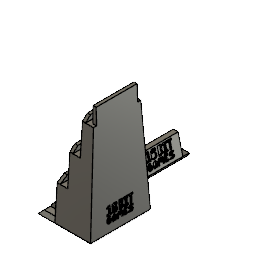
Nintendo DS Stand v8 (Autodesk Fusion 360 design; units mm, degrees)
Autodesk Fusion 360 part; units mm, degrees
(part 1 of 2)
sketch "Sketch1" plane through (0, 0, 0) normal (1, 0, 0) x (0, 0, -1)
  circle A0 centre (0, 0) radius 60
  line L0 (0.167, -59.9998) -> (20.167, -59.9998)
  line L1 (20.167, -59.9998) -> (20.167, -55)
  line L2 (20.167, -55) -> (-19.833, -55)
  line L3 (-19.833, -55) -> (-19.833, -59.9998)
  line L4 (-19.833, -59.9998) -> (20.167, -59.9998)
  line L5 (20.167, -59.9998) -> (20.167, -55)
  line L6 (20.167, -59.9998) -> (-19.833, -59.9998)
  line L7 (-19.833, -59.9998) -> (-19.833, -61.9998)
  line L8 (-19.833, -61.9998) -> (20.167, -61.9998)
  line L9 (20.167, -61.9998) -> (20.167, -59.9998)
  dimension "d1" = 120
  dimension "d2" = 20
  dimension "d3" = 40
  dimension "d4" = 2
  constraint coincident A0.centre origin
  constraint coincident A0 L0.start
  constraint horizontal L0
  constraint perpendicular L0 L1
  constraint horizontal L2
  constraint vertical L3
  constraint horizontal L4
  constraint vertical L5
  constraint horizontal L6
  constraint vertical L7
  constraint horizontal L8
  constraint vertical L9
  measures "d1" diameter of A0
  measures "d2" distance of L0.start L0.end
  measures "d3" distance of L1.end L2.end
  measures "d4" distance of L0.end L8.end
sketch "Sketch4" plane through (0, 0, 0) normal (1, 0, 0) x (0, 0, -1)
  line L0 (0, 0) -> (13, 0)
  line L1 (13, 0) -> (13, 10)
  line L2 (13, 10) -> (-13, 10)
  line L3 (-13, 10) -> (-13, 0)
  line L4 (-13, 0) -> (13, 0)
  line L5 (13, 0) -> (13, 10)
  dimension "d21" = 13
  dimension "d22" = 10
  dimension "d23" = 26
  dimension "d24" = 10
  constraint coincident L0.start origin
  constraint horizontal L0
  constraint perpendicular L0 L1
  constraint horizontal L2
  constraint vertical L3
  constraint horizontal L4
  constraint vertical L5
  measures "d21" distance of L0.start L0.end
  measures "d22" distance of L0.end L1.end
  measures "d23" distance of L1.end L2.end
  measures "d24" distance of L1.end L0.end
extrude "Extrude4" add sketch "Sketch4" along normal blind 2 makes body 1
sketch "Sketch5" plane through (2, 0, 0) normal (1, 0, 0) x (0, 0, -1)
  line L0 (13, 0) -> (13, 10)
  line L1 (13, 10) -> (-13, 10)
  line L2 (-13, 10) -> (-13, 0)
  line L3 (-13, 0) -> (13, 0)
  line L4 (-13, 0) -> (13, 0)
  line L5 (13, 0) -> (13, -2)
  line L6 (13, -2) -> (-13, -2)
  line L7 (-13, -2) -> (-13, 0)
  dimension "d27" = 2
  constraint horizontal L4
  constraint vertical L5
  constraint horizontal L6
  constraint vertical L7
  constraint coincident L2.end L3.start
  measures "d27" distance of L2.end L6.end
extrude "Extrude5" add sketch "Sketch5" along normal blind 2 separate body contours L3 L4 L5 L6 L7 makes body 2
extrude "Extrude6" add 1 faces at (2, -1.3333, -4.3333) along direction (-1, 0, 0) blind 3 on bodies 2 bodies 2 1
sketch "Sketch6" plane through (0, 0, 0) normal (0, 1, 0) x (-1, 0, 0)
  line L0 (0, 13) -> (0, -13)
  line L1 (0, -13) -> (1, -13)
  line L2 (1, -13) -> (1, 13)
  line L3 (1, 13) -> (0, 13)
  line L4 (1, 13) -> (3, 13)
  line L5 (3, 13) -> (3, -13)
  line L6 (3, -13) -> (1, -13)
  line L7 (1, -13) -> (1, 13)
  dimension "d32" = 2
  constraint horizontal L4
  constraint vertical L5
  constraint horizontal L6
  constraint vertical L7
  constraint coincident L2.end L3.start
  measures "d32" distance of L2.end L4.end
extrude "Extrude7" add sketch "Sketch6" along normal blind 3 separate body contours L2 L4 L5 L6 L7 makes body 3
extrude "Extrude8" add 1 faces at (-1, -1.3333, -4.3333) along direction (-1, 0, 0) blind 4 on bodies 2 bodies 2 3
sketch "Sketch7" plane through (0, 0, 13) normal (0, 0, 1) x (1, 0, 0)
  line L0 (-5, -2) -> (4, -2)
  line L1 (4, -2) -> (4, 0)
  line L2 (4, 0) -> (2, 0)
  line L3 (2, 0) -> (2, 10)
  line L4 (2, 10) -> (0, 10)
  line L5 (0, 10) -> (0, 0)
  line L6 (0, 0) -> (-1, 0)
  line L7 (-1, 0) -> (-1, 3)
  line L8 (-1, 3) -> (-3, 3)
  line L9 (-3, 3) -> (-3, 0)
  line L10 (-3, 0) -> (-5, 0)
  line L11 (-5, 0) -> (-5, -2)
  line L12 (-5, 0) -> (4, 0)
  line L13 (4, 0) -> (4, -2)
  line L14 (4, -2) -> (-5, -2)
  line L15 (-5, -2) -> (-5, 0)
  constraint horizontal L12
  constraint vertical L13
  constraint horizontal L14
  constraint vertical L15
  constraint coincident L0.end L1.start
  constraint coincident L10.end L11.start
extrude "Extrude9" add sketch "Sketch7" along normal blind 1 contours L0 L1 L2 L6 L10 L11 L12 L13 L14 L15 bodies 2
sketch "Sketch8" plane through (0, 0, -13) normal (0, 0, -1) x (-1, 0, 0)
  line L0 (5, 0) -> (3, 0)
  line L1 (3, 0) -> (3, 3)
  line L2 (3, 3) -> (1, 3)
  line L3 (1, 3) -> (1, 0)
  line L4 (1, 0) -> (0, 0)
  line L5 (0, 0) -> (0, 10)
  line L6 (0, 10) -> (-2, 10)
  line L7 (-2, 10) -> (-2, 0)
  line L8 (-2, 0) -> (-4, 0)
  line L9 (-4, 0) -> (-4, -2)
  line L10 (-4, -2) -> (5, -2)
  line L11 (5, -2) -> (5, 0)
  line L12 (-4, -2) -> (5, -2)
  line L13 (5, -2) -> (5, 0)
  line L14 (5, 0) -> (-4, 0)
  line L15 (-4, 0) -> (-4, -2)
  constraint horizontal L12
  constraint vertical L13
  constraint horizontal L14
  constraint vertical L15
  constraint coincident L0.start L11.end
  constraint coincident L9.end L10.start
extrude "Extrude10" add sketch "Sketch8" along normal blind 1 contours L0 L4 L8 L9 L10 L11 L12 L13 L14 L15 bodies 2
extrude "Extrude11" cut 1 faces at (4, -0.6667, -4.6667) along direction (-1, 0, 0) blind 1 on bodies 2 bodies 2
extrude "Extrude12" cut 1 faces at (-5, -1.3333, -4.6667) along direction (1, 0, 0) blind 1 on bodies 2 bodies 2
move_face "MoveFace1" by (-2, 0, 0) 3 faces at (-1, 2, -4.3333) (-3, 1, 4.3333) (-4, -1.3333, -4.6667) on bodies 2
draft "Draft5" angle 45 neutral plane through (-5, 0, -13) pull (0, 1, 0) 1 faces at (0, -0.6667, -14) on bodies 2
draft "Draft6" angle 45 neutral plane through (-5, 0, -13) pull (0, 1, 0) 1 faces at (-6, -1.3333, -5.3333) on bodies 2
draft "Draft7" angle 45 neutral plane through (-5, 0, -13) pull (0, 1, 0) 1 faces at (-3.6667, -1.3333, 14) on bodies 2
draft "Draft8" angle 45 neutral plane through (-5, 0, -13) pull (0, 1, 0) 1 faces at (3, -1.3333, -4.6667) on bodies 2
move_face "MoveFace5" by (0.4, 0, 0) 1 faces at (-3, 2, -4.3333) on bodies 2
extrude "Extrude13" cut 1 faces at (-2.6, 2, -4.3333) along direction (-1, 0, 0) blind 0.1 on bodies 2 bodies 2
extrude "Extrude14" add 1 faces at (0.6667, -2, 5.3333) along direction (0, -1, 0) blind 1 on bodies 2 bodies 2
sketch "Sketch9" plane through (0, 0, 0) normal (0, 1, 0) x (-1, 0, 0)
  line L0 (6, -14) -> (6, 14)
  line L1 (6, 14) -> (-3, 14)
  line L2 (-3, 14) -> (-3, -14)
  line L3 (-3, -14) -> (6, -14)
  line L4 (2.7, -13) -> (2.7, 13)
  line L5 (2.7, 13) -> (5, 13)
  line L6 (5, 13) -> (5, -13)
  line L7 (5, -13) -> (2.7, -13)
  line L8 (0, -13) -> (-2, -13)
  line L9 (-2, -13) -> (-2, 13)
  line L10 (-2, 13) -> (0, 13)
  line L11 (0, 13) -> (0, -13)
draft "Draft9" angle 14 neutral plane through (0, 10, -13) pull (0, 1, 0) 1 faces at (2, 3.3333, -4.3333) on bodies 2
draft "Draft10" angle 30.9 neutral plane through (0, 3, 0) pull (0, 1, 0) 1 faces at (-5, 2, 4.3333) on bodies 2
move_face "MoveFace6" by (0, 0, -1) 2 faces at (0.6667, -2.3333, -16) (-3, -1.3333, -15.3333) on bodies 2
move_face "MoveFace7" by (0, 0, 1) 2 faces at (0.6667, -2.6667, 16) (-3, -1.3333, 15.3333) on bodies 2
move_face "MoveFace8" by (1, 0, 0) 3 faces at (5, -2.6667, -5.6667) (3.9928, 2.0072, 4.3333) (4.3298, -1.3298, -15) on bodies 2
move_face "MoveFace9" by (-1, 0, 0) 3 faces at (-8, -2.3333, 4.3333) (-6.9874, -0.3208, -4.3333) (-7.3271, -1.3271, 15) on bodies 2
extrude "Extrude15" add 1 faces at (-5.2333, 1, 13) along direction (0, 0, 1) blind 2 on bodies 2 bodies 2
extrude "Extrude16" add 1 faces at (-5.2333, 1, -13) along direction (0, 0, -1) blind 2 on bodies 2 bodies 2
move_face "MoveFace10" by (-0.1, 0, 0) 1 faces at (-2.7, 2, 5) on bodies 2
move_face "MoveFace11" by (0.1, 0, 0) 1 faces at (0, 3.3333, -4.3333) on bodies 2
move_face "MoveFace12" by (0.1, 0, 0) 1 faces at (-2.8, 1, -5) on bodies 2
move_face "MoveFace13" by (-0.05, 0, 0) 1 faces at (0.1, 3.3333, -4.3333) on bodies 2
sketch "Sketch10" plane through (5.1718, 1.2895, 0) normal (0.970296, 0.241922, 0) x (0, 0, -1)
  line L0 (13, -3.3791) -> (13, 8.9772)
  line L1 (13, 8.9772) -> (-13, 8.9772)
  line L2 (-13, 8.9772) -> (-13, -3.3791)
  line L3 (-13, -3.3791) -> (13, -3.3791)
  line L4 (93, 16) -> (93, 15)
  line L5 (96, 16) -> (96, 17)
  line L6 (93, 18) -> (97, 18)
  line L7 (98, 15) -> (97, 15)
  line L8 (98, 14) -> (98, 15)
  line L9 (97, 17) -> (98, 17)
  line L10 (94, 17) -> (94, 16)
  line L11 (93, 17) -> (93, 18)
  line L12 (92, 15) -> (92, 14)
  line L13 (91, 14) -> (91, 15)
  line L14 (90, 15) -> (90, 16)
  line L15 (86, 18) -> (90, 18)
  line L16 (89, 14) -> (90, 14)
  line L17 (92, 16) -> (92, 17)
  line L18 (93, 15) -> (92, 15)
  line L19 (90, 18) -> (90, 17)
  line L20 (91, 17) -> (91, 16)
  line L21 (92, 17) -> (93, 17)
  line L22 (55, 46) -> (54, 46)
  line L23 (50, 0) -> (50, 4)
  line L24 (57, 43) -> (56, 43)
  line L25 (130, 7) -> (130, 8)
  line L26 (54, 2) -> (55, 2)
  line L27 (73, 12) -> (73, 13)
  line L28 (53, 47) -> (53, 46)
  line L29 (74, 13) -> (74, 12)
  line L30 (78, 13) -> (77, 13)
  line L31 (52, 3) -> (52, 2)
  line L32 (70, 46) -> (70, 45)
  line L33 (87, 13) -> (87, 12)
  line L34 (50, 4) -> (51, 4)
  line L35 (132, 2) -> (131, 2)
  line L36 (78, 1) -> (78, 13)
  line L37 (75, 5) -> (72, 5)
  line L38 (69, 44) -> (68, 44)
  line L39 (54, 46) -> (54, 45)
  line L40 (50, 48) -> (54, 48)
  line L41 (54, 45) -> (53, 45)
  line L42 (56, 5) -> (55, 5)
  line L43 (54, 47) -> (53, 47)
  line L44 (55, 5) -> (55, 6)
  line L45 (72, 4) -> (75, 4)
  line L46 (75, 12) -> (75, 7)
  line L47 (83, 13) -> (83, 1)
  line L48 (51, 4) -> (51, 3)
  line L49 (52, 43) -> (56, 43)
  line L50 (79, 0) -> (82, 0)
  line L51 (54, 5) -> (53, 5)
  line L52 (131, 3) -> (131, 4)
  line L53 (53, 4) -> (53, 3)
  line L54 (51, 44) -> (50, 44)
  line L55 (86, 13) -> (86, 14)
  line L56 (69, 13) -> (69, 1)
  line L57 (68, 0) -> (68, 14)
  line L58 (87, 12) -> (86, 12)
  line L59 (51, 45) -> (51, 44)
  line L60 (55, 47) -> (55, 46)
  line L61 (51, 5) -> (52, 5)
  line L62 (53, 44) -> (52, 44)
  line L63 (131, 1) -> (130, 1)
  line L64 (53, 1) -> (54, 1)
  line L65 (56, 4) -> (56, 5)
  line L66 (75, 13) -> (75, 14)
  line L67 (50, 42) -> (56, 42)
  line L68 (133, 3) -> (132, 3)
  line L69 (55, 2) -> (55, 1)
  line L70 (85, 13) -> (86, 13)
  line L71 (69, 47) -> (70, 47)
  line L72 (72, 12) -> (73, 12)
  line L73 (132, 15) -> (132, 17)
  line L74 (53, 45) -> (53, 44)
  line L75 (52, 45) -> (51, 45)
  line L76 (52, 44) -> (52, 43)
  line L77 (71, 5) -> (71, 1)
  line L78 (72, 5) -> (71, 5)
  line L79 (71, 6) -> (76, 6)
  line L80 (72, 0) -> (72, 4)
  line L81 (69, 1) -> (71, 1)
  line L82 (86, 12) -> (86, 0)
  line L83 (83, 1) -> (85, 1)
  line L84 (76, 1) -> (76, 5)
  line L85 (74, 12) -> (75, 12)
  line L86 (75, 4) -> (75, 0)
  line L87 (75, 5) -> (76, 5)
  line L88 (78, 1) -> (76, 1)
  line L89 (108, 4) -> (115, 4)
  line L90 (100, 13) -> (99, 13)
  line L91 (104, 48) -> (104, 43)
  line L92 (100, 15) -> (100, 14)
  line L93 (120, 43) -> (124, 43)
  line L94 (71, 22) -> (80, 22)
  line L95 (97, 27) -> (97, 33)
  line L96 (109, 44) -> (109, 26)
  line L97 (73, 25) -> (73, 26)
  line L98 (78, 27) -> (78, 26)
  line L99 (105, 26) -> (105, 23)
  line L100 (104, 18) -> (115, 18)
  line L101 (107, 15) -> (114, 15)
  line L102 (86, 15) -> (85, 15)
  line L103 (82, 14) -> (83, 14)
  line L104 (108, 11) -> (111, 11)
  line L105 (113, 44) -> (117, 44)
  line L106 (105, 17) -> (105, 1)
  line L107 (52, 15) -> (51, 15)
  line L108 (133, 43) -> (133, 48)
  line L109 (71, 32) -> (72, 32)
  line L110 (98, 25) -> (98, 24)
  line L111 (132, 47) -> (132, 44)
  line L112 (125, 23) -> (128, 23)
  line L113 (117, 47) -> (105, 47)
  line L114 (89, 48) -> (89, 22)
  line L115 (108, 27) -> (108, 43)
  line L116 (104, 0) -> (104, 18)
  line L117 (84, 14) -> (84, 13)
  line L118 (81, 24) -> (82, 24)
  line L119 (79, 47) -> (71, 47)
  line L120 (63, 4) -> (63, 10)
  line L121 (85, 14) -> (84, 14)
  line L122 (132, 43) -> (133, 43)
  line L123 (114, 3) -> (107, 3)
  line L124 (105, 1) -> (114, 1)
  line L125 (105, 44) -> (109, 44)
  line L126 (85, 15) -> (85, 14)
  line L127 (100, 26) -> (100, 33)
  line L128 (83, 14) -> (83, 15)
  line L129 (85, 17) -> (86, 17)
  line L130 (55, 15) -> (60, 15)
  line L131 (104, 22) -> (104, 27)
  line L132 (82, 0) -> (82, 14)
  line L133 (74, 26) -> (76, 26)
  line L134 (101, 0) -> (104, 0)
  line L135 (58, 10) -> (58, 8)
  line L136 (111, 7) -> (108, 7)
  line L137 (60, 17) -> (55, 17)
  line L138 (80, 23) -> (81, 23)
  line L139 (125, 23) -> (125, 44)
  line L140 (84, 16) -> (85, 16)
  line L141 (77, 27) -> (76, 27)
  line L142 (99, 25) -> (98, 25)
  line L143 (99, 14) -> (98, 14)
  line L144 (73, 13) -> (74, 13)
  line L145 (51, 15) -> (51, 14)
  line L146 (98, 1) -> (100, 1)
  line L147 (77, 25) -> (73, 25)
  line L148 (83, 15) -> (84, 15)
  line L149 (98, 16) -> (99, 16)
  line L150 (104, 27) -> (108, 27)
  line L151 (72, 14) -> (72, 13)
  line L152 (85, 16) -> (85, 17)
  line L153 (114, 17) -> (105, 17)
  line L154 (99, 35) -> (99, 36)
  line L155 (117, 26) -> (113, 26)
  line L156 (124, 43) -> (124, 22)
  line L157 (84, 15) -> (84, 16)
  line L158 (72, 27) -> (71, 27)
  line L159 (54, 13) -> (54, 14)
  line L160 (121, 44) -> (121, 47)
  line L161 (90, 23) -> (90, 47)
  line L162 (55, 16) -> (54, 16)
  line L163 (118, 27) -> (114, 27)
  line L164 (121, 47) -> (132, 47)
  line L165 (78, 26) -> (77, 26)
  line L166 (101, 34) -> (100, 34)
  line L167 (73, 27) -> (73, 28)
  line L168 (117, 23) -> (117, 26)
  line L169 (54, 14) -> (55, 14)
  line L170 (114, 43) -> (118, 43)
  line L171 (129, 43) -> (132, 43)
  line L172 (99, 24) -> (100, 24)
  line L173 (99, 33) -> (100, 33)
  line L174 (98, 34) -> (99, 34)
  line L175 (86, 16) -> (86, 15)
  line L176 (54, 15) -> (53, 15)
  line L177 (80, 25) -> (81, 25)
  line L178 (120, 43) -> (120, 48)
  line L179 (133, 48) -> (132, 48)
  line L180 (98, 17) -> (98, 16)
  line L181 (94, 16) -> (93, 16)
  line L182 (91, 16) -> (92, 16)
  line L183 (89, 15) -> (89, 14)
  line L184 (92, 14) -> (91, 14)
  line L185 (50, 0) -> (133, 0)
  line L186 (90, 16) -> (89, 16)
  line L187 (89, 16) -> (89, 17)
  line L188 (87, 15) -> (89, 15)
  line L189 (97, 18) -> (97, 17)
  line L190 (123, 10) -> (123, 9)
  line L191 (128, 6) -> (127, 6)
  line L192 (61, 0) -> (61, 1)
  line L193 (62, 3) -> (62, 4)
  line L194 (70, 14) -> (70, 13)
  line L195 (69, 45) -> (69, 44)
  line L196 (50, 44) -> (50, 42)
  line L197 (72, 7) -> (72, 12)
  line L198 (133, 14) -> (124, 14)
  line L199 (61, 3) -> (62, 3)
  line L200 (71, 46) -> (70, 46)
  line L201 (52, 2) -> (53, 2)
  line L202 (54, 4) -> (54, 5)
  line L203 (70, 45) -> (69, 45)
  line L204 (77, 43) -> (77, 42)
  line L205 (60, 47) -> (55, 47)
  line L206 (50, 0) -> (50, 1)
  line L207 (129, 10) -> (130, 10)
  line L208 (59, 5) -> (59, 4)
  line L209 (68, 45) -> (68, 46)
  line L210 (61, 1) -> (62, 1)
  line L211 (79, 35) -> (79, 36)
  line L212 (131, 4) -> (132, 4)
  line L213 (124, 11) -> (123, 11)
  line L214 (52, 5) -> (52, 4)
  line L215 (54, 3) -> (54, 2)
  line L216 (124, 14) -> (124, 12)
  line L217 (61, 0) -> (62, 0)
  line L218 (73, 42) -> (74, 42)
  line L219 (85, 1) -> (85, 13)
  line L220 (53, 2) -> (53, 1)
  line L221 (129, 4) -> (129, 3)
  line L222 (69, 46) -> (69, 47)
  line L223 (128, 10) -> (124, 10)
  line L224 (79, 36) -> (78, 36)
  line L225 (123, 11) -> (123, 12)
  line L226 (133, 18) -> (133, 14)
  line L227 (53, 46) -> (52, 46)
  line L228 (71, 13) -> (71, 6)
  line L229 (125, 11) -> (129, 11)
  line L230 (131, 8) -> (132, 8)
  line L231 (71, 35) -> (71, 42)
  line L232 (52, 46) -> (52, 45)
  line L233 (61, 2) -> (61, 3)
  line L234 (130, 4) -> (129, 4)
  line L235 (76, 13) -> (75, 13)
  line L236 (55, 3) -> (55, 4)
  line L237 (70, 47) -> (70, 48)
  line L238 (124, 10) -> (124, 11)
  line L239 (73, 36) -> (73, 35)
  line L240 (53, 3) -> (54, 3)
  line L241 (130, 9) -> (131, 9)
  line L242 (123, 17) -> (123, 16)
  line L243 (60, 1) -> (60, 2)
  line L244 (55, 6) -> (54, 6)
  line L245 (72, 41) -> (73, 41)
  line L246 (54, 1) -> (54, 0)
  line L247 (54, 48) -> (54, 47)
  line L248 (75, 7) -> (72, 7)
  line L249 (52, 4) -> (53, 4)
  line L250 (55, 1) -> (60, 1)
  line L251 (69, 24) -> (70, 24)
  line L252 (71, 17) -> (72, 17)
  line L253 (100, 38) -> (99, 38)
  line L254 (74, 33) -> (76, 33)
  line L255 (74, 43) -> (77, 43)
  line L256 (119, 4) -> (128, 4)
  line L257 (70, 16) -> (71, 16)
  line L258 (62, 5) -> (61, 5)
  line L259 (99, 36) -> (100, 36)
  line L260 (72, 16) -> (72, 15)
  line L261 (96, 39) -> (96, 38)
  line L262 (130, 8) -> (129, 8)
  line L263 (78, 37) -> (74, 37)
  line L264 (62, 1) -> (62, 2)
  line L265 (77, 34) -> (77, 33)
  line L266 (72, 43) -> (73, 43)
  line L267 (92, 34) -> (92, 26)
  line L268 (76, 33) -> (76, 32)
  line L269 (96, 26) -> (96, 27)
  line L270 (72, 15) -> (71, 15)
  line L271 (92, 45) -> (96, 45)
  line L272 (95, 40) -> (95, 39)
  line L273 (78, 42) -> (78, 41)
  line L274 (70, 23) -> (71, 23)
  line L275 (114, 15) -> (114, 17)
  line L276 (131, 2) -> (131, 1)
  line L277 (73, 16) -> (72, 16)
  line L278 (115, 18) -> (115, 14)
  line L279 (64, 26) -> (60, 26)
  line L280 (83, 45) -> (82, 45)
  line L281 (82, 41) -> (82, 44)
  line L282 (120, 12) -> (121, 12)
  line L283 (54, 0) -> (61, 0)
  line L284 (70, 26) -> (70, 25)
  line L285 (81, 45) -> (80, 45)
  line L286 (64, 23) -> (64, 26)
  line L287 (72, 37) -> (72, 41)
  line L288 (83, 40) -> (83, 45)
  line L289 (120, 15) -> (120, 16)
  line L290 (89, 22) -> (98, 22)
  line L291 (80, 47) -> (80, 48)
  line L292 (131, 7) -> (130, 7)
  line L293 (72, 32) -> (72, 33)
  line L294 (96, 45) -> (96, 44)
  line L295 (61, 4) -> (60, 4)
  line L296 (99, 47) -> (99, 48)
  line L297 (73, 15) -> (73, 14)
  line L298 (76, 6) -> (76, 13)
  line L299 (99, 37) -> (96, 37)
  line L300 (82, 35) -> (81, 35)
  line L301 (61, 27) -> (61, 48)
  line L302 (72, 31) -> (73, 31)
  line L303 (132, 3) -> (132, 2)
  line L304 (73, 14) -> (72, 14)
  line L305 (77, 42) -> (78, 42)
  line L306 (129, 6) -> (130, 6)
  line L307 (78, 33) -> (78, 32)
  line L308 (57, 7) -> (61, 7)
  line L309 (73, 37) -> (72, 37)
  line L310 (128, 7) -> (129, 7)
  line L311 (67, 27) -> (67, 26)
  line L312 (79, 41) -> (79, 43)
  line L313 (128, 4) -> (128, 6)
  line L314 (71, 15) -> (71, 14)
  line L315 (83, 34) -> (82, 34)
  line L316 (62, 4) -> (63, 4)
  line L317 (81, 33) -> (81, 34)
  line L318 (129, 7) -> (129, 6)
  line L319 (74, 32) -> (74, 33)
  line L320 (98, 46) -> (99, 46)
  line L321 (130, 2) -> (130, 3)
  line L322 (70, 24) -> (70, 23)
  line L323 (74, 36) -> (73, 36)
  line L324 (69, 15) -> (70, 15)
  line L325 (77, 31) -> (78, 31)
  line L326 (132, 4) -> (132, 6)
  line L327 (79, 37) -> (79, 38)
  line L328 (78, 32) -> (79, 32)
  line L329 (50, 27) -> (50, 26.9)
  line L330 (122, 10) -> (123, 10)
  line L331 (72, 17) -> (72, 18)
  line L332 (73, 31) -> (73, 32)
  line L333 (77, 33) -> (78, 33)
  line L334 (96, 38) -> (92, 38)
  line L335 (123, 9) -> (124, 9)
  line L336 (60, 5) -> (59, 5)
  line L337 (67, 27) -> (67, 45)
  line L338 (130, 6) -> (130, 4)
  line L339 (78, 36) -> (78, 37)
  line L340 (79, 38) -> (73, 38)
  line L341 (59, 4) -> (56, 4)
  line L342 (60, 2) -> (61, 2)
  line L343 (60, 4) -> (60, 3)
  line L344 (79, 32) -> (78, 32)
  line L345 (123, 14) -> (123, 15)
  line L346 (72, 42) -> (72, 43)
  line L347 (67, 45) -> (68, 45)
  line L348 (127, 6) -> (127, 7)
  line L349 (122, 14) -> (123, 14)
  line L350 (68, 26) -> (68, 25)
  line L351 (132, 7) -> (133, 7)
  line L352 (60, 3) -> (55, 3)
  line L353 (78, 43) -> (79, 43)
  line L354 (78, 41) -> (78, 40)
  line L355 (63, 3) -> (64, 3)
  line L356 (54, 0) -> (61, 0)
  line L357 (71, 16) -> (71, 17)
  line L358 (68, 14) -> (69, 14)
  line L359 (70, 25) -> (71, 25)
  line L360 (61, 5) -> (61, 4)
  line L361 (129, 9) -> (128, 9)
  line L362 (73, 38) -> (73, 37)
  line L363 (128, 8) -> (128, 7)
  line L364 (124, 8) -> (128, 8)
  line L365 (73, 44) -> (78, 44)
  line L366 (73, 31) -> (72, 31)
  line L367 (69, 14) -> (69, 15)
  line L368 (81, 34) -> (80, 34)
  line L369 (73, 33) -> (73, 34)
  line L370 (74, 37) -> (74, 36)
  line L371 (77, 32) -> (77, 31)
  line L372 (63, 2) -> (63, 3)
  line L373 (123, 15) -> (132, 15)
  line L374 (78, 44) -> (78, 43)
  line L375 (61, 6) -> (60, 6)
  line L376 (129, 11) -> (129, 10)
  line L377 (132, 8) -> (132, 7)
  line L378 (82, 33) -> (81, 33)
  line L379 (129, 1) -> (129, 2)
  line L380 (72, 18) -> (75, 18)
  line L381 (73, 34) -> (77, 34)
  line L382 (72, 13) -> (71, 13)
  line L383 (132, 6) -> (131, 6)
  line L384 (128, 9) -> (128, 10)
  line L385 (74, 15) -> (73, 15)
  line L386 (129, 2) -> (130, 2)
  line L387 (61, 7) -> (61, 6)
  line L388 (73, 32) -> (74, 32)
  line L389 (62, 2) -> (63, 2)
  line L390 (51, 3) -> (52, 3)
  line L391 (73, 17) -> (73, 16)
  line L392 (123, 12) -> (122, 12)
  line L393 (72, 33) -> (73, 33)
  line L394 (130, 3) -> (131, 3)
  line L395 (55, 4) -> (54, 4)
  line L396 (79, 46) -> (79, 47)
  line L397 (76, 32) -> (77, 32)
  line L398 (74, 42) -> (74, 43)
  line L399 (125, 12) -> (125, 11)
  line L400 (130, 1) -> (130, 0)
  line L401 (73, 43) -> (73, 44)
  line L402 (73, 41) -> (73, 42)
  line L403 (60, 6) -> (60, 5)
  line L404 (133, 7) -> (133, 3)
  line L405 (123, 16) -> (122, 16)
  line L406 (131, 6) -> (131, 7)
  line L407 (130, 10) -> (130, 9)
  line L408 (71, 47) -> (71, 46)
  line L409 (57, 42) -> (57, 43)
  line L410 (68, 46) -> (69, 46)
  line L411 (74, 17) -> (73, 17)
  line L412 (132, 17) -> (123, 17)
  line L413 (124, 12) -> (125, 12)
  line L414 (82, 34) -> (82, 35)
  line L415 (98, 24) -> (97, 24)
  line L416 (98, 35) -> (98, 34)
  line L417 (73, 28) -> (72, 28)
  line L418 (72, 23) -> (79, 23)
  line L419 (100, 26) -> (99, 26)
  line L420 (51, 13) -> (51, 5)
  line L421 (98, 23) -> (99, 23)
  line L422 (129, 8) -> (129, 9)
  line L423 (118, 22) -> (118, 27)
  line L424 (53, 16) -> (52, 16)
  line L425 (81, 25) -> (81, 26)
  line L426 (52, 16) -> (52, 15)
  line L427 (81, 23) -> (81, 24)
  line L428 (132, 44) -> (128, 44)
  line L429 (104, 22) -> (118, 22)
  line L430 (80, 34) -> (80, 35)
  line L431 (101, 25) -> (101, 34)
  line L432 (100, 47) -> (99, 47)
  line L433 (76, 17) -> (76, 16)
  line L434 (60, 26) -> (60, 47)
  line L435 (113, 26) -> (113, 44)
  line L436 (100, 25) -> (101, 25)
  line L437 (52, 13) -> (51, 13)
  line L438 (128, 23) -> (125, 23)
  line L439 (87, 16) -> (86, 16)
  line L440 (54, 18) -> (54, 17)
  line L441 (99, 34) -> (99, 33)
  line L442 (86, 17) -> (86, 18)
  line L443 (54, 16) -> (54, 15)
  line L444 (53, 14) -> (52, 14)
  line L445 (124, 22) -> (129, 22)
  line L446 (77, 14) -> (76, 14)
  line L447 (105, 23) -> (117, 23)
  line L448 (57, 42) -> (57, 27)
  line L449 (58, 8) -> (62, 8)
  line L450 (77, 28) -> (77, 27)
  line L451 (131, 9) -> (131, 8)
  line L452 (129, 22) -> (129, 43)
  line L453 (73, 26) -> (72, 26)
  line L454 (98, 47) -> (98, 46)
  line L455 (105, 47) -> (105, 44)
  line L456 (98, 22) -> (98, 23)
  line L457 (56, 13) -> (56, 14)
  line L458 (79, 23) -> (79, 24)
  line L459 (128, 44) -> (128, 23)
  line L460 (118, 43) -> (118, 48)
  line L461 (125, 44) -> (121, 44)
  line L462 (54, 17) -> (53, 17)
  line L463 (108, 43) -> (104, 43)
  line L464 (109, 26) -> (105, 26)
  line L465 (80, 22) -> (80, 23)
  line L466 (117, 44) -> (117, 47)
  line L467 (64, 3) -> (64, 11)
  line L468 (100, 35) -> (99, 35)
  line L469 (96, 27) -> (97, 27)
  line L470 (121, 12) -> (121, 11)
  line L471 (114, 27) -> (114, 43)
  line L472 (82, 25) -> (83, 25)
  line L473 (53, 15) -> (53, 14)
  line L474 (77, 16) -> (77, 15)
  line L475 (121, 10) -> (120, 10)
  line L476 (96, 40) -> (95, 40)
  line L477 (60, 15) -> (60, 17)
  line L478 (76, 14) -> (76, 15)
  line L479 (123, 8) -> (122, 8)
  line L480 (83, 25) -> (83, 34)
  line L481 (57, 26) -> (51, 26)
  line L482 (124, 9) -> (124, 8)
  line L483 (93, 39) -> (95, 39)
  line L484 (122, 16) -> (122, 15)
  line L485 (78, 15) -> (78, 14)
  line L486 (82, 26) -> (82, 33)
  line L487 (120, 14) -> (120, 12)
  line L488 (75, 15) -> (75, 16)
  line L489 (71, 25) -> (71, 24)
  line L490 (121, 17) -> (122, 17)
  line L491 (53, 17) -> (53, 16)
  line L492 (97, 35) -> (98, 35)
  line L493 (72, 26) -> (72, 27)
  line L494 (53, 5) -> (53, 13)
  line L495 (79, 41) -> (82, 41)
  line L496 (120, 10) -> (120, 11)
  line L497 (75, 14) -> (74, 14)
  line L498 (122, 11) -> (122, 10)
  line L499 (122, 8) -> (122, 9)
  line L500 (78, 28) -> (77, 28)
  line L501 (93, 39) -> (93, 44)
  line L502 (61, 14) -> (61, 18)
  line L503 (68, 27) -> (69, 27)
  line L504 (79, 14) -> (79, 0)
  line L505 (51, 23) -> (64, 23)
  line L506 (78, 31) -> (78, 28)
  line L507 (51, 14) -> (50, 14)
  line L508 (96, 37) -> (96, 36)
  line L509 (74, 26) -> (74, 27)
  line L510 (99, 45) -> (100, 45)
  line L511 (100, 24) -> (100, 25)
  line L512 (99, 26) -> (99, 25)
  line L513 (65, 27) -> (61, 27)
  line L514 (52, 14) -> (52, 13)
  line L515 (97, 39) -> (96, 39)
  line L516 (74, 27) -> (73, 27)
  line L517 (97, 24) -> (97, 23)
  line L518 (68, 44) -> (68, 27)
  line L519 (95, 44) -> (95, 43)
  line L520 (76, 15) -> (75, 15)
  line L521 (80, 35) -> (79, 35)
  line L522 (97, 23) -> (90, 23)
  line L523 (78, 14) -> (79, 14)
  line L524 (96, 44) -> (97, 44)
  line L525 (75, 16) -> (74, 16)
  line L526 (96, 36) -> (97, 36)
  line L527 (122, 9) -> (121, 9)
  line L528 (72, 24) -> (72, 23)
  line L529 (63, 10) -> (58, 10)
  line L530 (56, 42) -> (56, 27)
  line L531 (73, 26) -> (73, 25)
  line L532 (99, 23) -> (99, 24)
  line L533 (97, 33) -> (96, 33)
  line L534 (100, 34) -> (100, 35)
  line L535 (100, 45) -> (100, 38)
  line L536 (121, 16) -> (121, 17)
  line L537 (76, 16) -> (77, 16)
  line L538 (120, 3) -> (120, 1)
  line L539 (127, 7) -> (123, 7)
  line L540 (129, 3) -> (120, 3)
  line L541 (122, 15) -> (121, 15)
  line L542 (55, 13) -> (56, 13)
  line L543 (51, 26) -> (51, 23)
  line L544 (75, 18) -> (75, 17)
  line L545 (95, 43) -> (96, 43)
  line L546 (95, 44) -> (93, 44)
  line L547 (96, 33) -> (96, 34)
  line L548 (96, 28) -> (95, 28)
  line L549 (69, 27) -> (69, 26)
  line L550 (101, 37) -> (101, 46)
  line L551 (100, 36) -> (100, 37)
  line L552 (82, 24) -> (82, 25)
  line L553 (115, 0) -> (119, 0)
  line L554 (74, 14) -> (74, 15)
  line L555 (53, 13) -> (54, 13)
  line L556 (78, 40) -> (83, 40)
  line L557 (55, 14) -> (55, 15)
  line L558 (114, 1) -> (114, 3)
  line L559 (76, 27) -> (76, 26)
  line L560 (92, 26) -> (96, 26)
  line L561 (79, 24) -> (79, 23)
  line L562 (50, 27) -> (50, 22)
  line L563 (122, 14) -> (122, 12)
  line L564 (80, 45) -> (80, 46)
  line L565 (93, 33) -> (95, 33)
  line L566 (80, 37) -> (79, 37)
  line L567 (65, 22) -> (65, 27)
  line L568 (97, 44) -> (97, 39)
  line L569 (75, 17) -> (76, 17)
  line L570 (77, 15) -> (78, 15)
  line L571 (77, 26) -> (77, 25)
  line L572 (84, 13) -> (83, 13)
  line L573 (121, 11) -> (122, 11)
  line L574 (64, 11) -> (57, 11)
  line L575 (69, 25) -> (69, 24)
  line L576 (79, 35) -> (80, 35)
  line L577 (67, 26) -> (68, 26)
  line L578 (55, 17) -> (55, 16)
  line L579 (120, 1) -> (129, 1)
  line L580 (92, 39) -> (92, 45)
  line L581 (119, 4) -> (119, 0)
  line L582 (96, 43) -> (96, 40)
  line L583 (123, 7) -> (123, 8)
  line L584 (61, 18) -> (54, 18)
  line L585 (70, 13) -> (69, 13)
  line L586 (119, 15) -> (120, 15)
  line L587 (80, 46) -> (79, 46)
  line L588 (74, 16) -> (74, 17)
  line L589 (56, 14) -> (61, 14)
  line L590 (81, 26) -> (82, 26)
  line L591 (115, 4) -> (115, 0)
  line L592 (55, 12) -> (55, 13)
  line L593 (120, 11) -> (119, 11)
  line L594 (71, 23) -> (71, 22)
  line L595 (72, 28) -> (72, 31)
  line L596 (79, 24) -> (80, 24)
  line L597 (95, 28) -> (95, 27)
  line L598 (81, 35) -> (81, 36)
  line L599 (54, 6) -> (54, 12)
  line L600 (100, 46) -> (100, 47)
  line L601 (96, 32) -> (96, 28)
  line L602 (95, 33) -> (95, 32)
  line L603 (121, 9) -> (121, 10)
  line L604 (82, 45) -> (82, 46)
  line L605 (69, 26) -> (70, 26)
  line L606 (71, 14) -> (70, 14)
  line L607 (57, 27) -> (57, 26)
  line L608 (79, 32) -> (79, 27)
  line L609 (81, 36) -> (80, 36)
  line L610 (93, 27) -> (95, 27)
  line L611 (121, 14) -> (120, 14)
  line L612 (50, 22) -> (65, 22)
  line L613 (99, 46) -> (99, 45)
  line L614 (80, 24) -> (80, 25)
  line L615 (101, 46) -> (100, 46)
  line L616 (79, 27) -> (78, 27)
  line L617 (68, 25) -> (69, 25)
  line L618 (82, 46) -> (81, 46)
  line L619 (120, 16) -> (121, 16)
  line L620 (99, 38) -> (99, 37)
  line L621 (121, 15) -> (121, 14)
  line L622 (100, 37) -> (101, 37)
  line L623 (80, 36) -> (80, 37)
  line L624 (56, 27) -> (50, 27)
  line L625 (133, 18) -> (122, 18)
  line L626 (119, 11) -> (119, 15)
  line L627 (92, 38) -> (92, 39)
  line L628 (95, 32) -> (96, 32)
  line L629 (54, 12) -> (55, 12)
  line L630 (90, 47) -> (98, 47)
  line L631 (81, 46) -> (81, 47)
  line L632 (93, 27) -> (93, 33)
  line L633 (122, 17) -> (122, 18)
  line L634 (81, 47) -> (80, 47)
  line L635 (71, 27) -> (71, 32)
  line L636 (81, 44) -> (81, 45)
  line L637 (82, 44) -> (81, 44)
  line L638 (70, 15) -> (70, 16)
  line L639 (96, 34) -> (92, 34)
  line L640 (77, 13) -> (77, 14)
  line L641 (71, 24) -> (72, 24)
  line L642 (107, 3) -> (107, 8)
  line L643 (100, 14) -> (101, 14)
  line L644 (133, 0) -> (133, 48)
  line L645 (107, 10) -> (107, 15)
  line L646 (50, 48) -> (50, 0)
  line L647 (108, 14) -> (108, 11)
  line L648 (99, 13) -> (99, 14)
  line L649 (61, 0) -> (68, 0)
  line L650 (101, 14) -> (101, 0)
  line L651 (97, 36) -> (97, 35)
  line L652 (87, 17) -> (87, 16)
  line L653 (107, 8) -> (110, 8)
  line L654 (57, 11) -> (57, 7)
  line L655 (100, 1) -> (100, 13)
  line L656 (73, 35) -> (71, 35)
  line L657 (111, 11) -> (111, 7)
  line L658 (110, 10) -> (107, 10)
  line L659 (108, 7) -> (108, 4)
  line L660 (87, 14) -> (87, 15)
  line L661 (99, 16) -> (99, 15)
  line L662 (86, 14) -> (87, 14)
  line L663 (62, 8) -> (62, 5)
  line L664 (71, 42) -> (72, 42)
  line L665 (99, 48) -> (104, 48)
  line L666 (110, 8) -> (110, 10)
  line L667 (115, 14) -> (108, 14)
  line L668 (99, 15) -> (100, 15)
  line L669 (94, 12) -> (93, 12)
  line L670 (90, 12) -> (89, 12)
  line L671 (97, 0) -> (97, 12)
  line L672 (97, 16) -> (96, 16)
  line L673 (93, 12) -> (93, 7)
  line L674 (93, 7) -> (90, 7)
  line L675 (90, 7) -> (90, 12)
  line L676 (91, 8) -> (92, 8)
  line L677 (97, 12) -> (96, 12)
  line L678 (89, 12) -> (89, 13)
  line L679 (97, 14) -> (97, 13)
  line L680 (96, 12) -> (96, 13)
  line L681 (90, 13) -> (91, 13)
  line L682 (98, 13) -> (98, 1)
  line L683 (97, 13) -> (98, 13)
  line L684 (91, 13) -> (91, 8)
  line L685 (92, 13) -> (93, 13)
  line L686 (90, 14) -> (90, 13)
  line L687 (94, 13) -> (94, 12)
  line L688 (96, 13) -> (94, 13)
  line L689 (93, 13) -> (93, 14)
  line L690 (92, 8) -> (92, 13)
  line L691 (94, 15) -> (96, 15)
  line L692 (97, 15) -> (97, 16)
  line L693 (94, 14) -> (94, 15)
  line L694 (96, 14) -> (97, 14)
  line L695 (93, 14) -> (94, 14)
  line L696 (133, 48) -> (50, 48)
  line L697 (96, 17) -> (94, 17)
  line L698 (91, 15) -> (90, 15)
  line L699 (89, 17) -> (87, 17)
  line L700 (80, 48) -> (89, 48)
  line L701 (89, 13) -> (87, 13)
  line L702 (90, 17) -> (91, 17)
  line L703 (96, 15) -> (96, 14)
  point P0 (50, 0)
  dimension "d65" = 4
  dimension "d66" = 1
  dimension "d67" = 1
  dimension "d68" = 1
  dimension "d69" = 1
  dimension "d70" = 1
  dimension "d71" = 1
  dimension "d72" = 1
  dimension "d73" = 2
  dimension "d74" = 6
  dimension "d75" = 15
  dimension "d76" = 5
  dimension "d77" = 1
  dimension "d78" = 6
  dimension "d79" = 15
  dimension "d80" = 5
  dimension "d81" = 4
  dimension "d82" = 3
  dimension "d83" = 5
  constraint perpendicular L43 L247
  constraint perpendicular L28 L43
  constraint perpendicular L28 L227
  constraint perpendicular L227 L232
  constraint perpendicular L75 L232
  constraint perpendicular L59 L75
  constraint perpendicular L54 L196
  constraint perpendicular L67 L530
  constraint perpendicular L562 L624
  constraint perpendicular L481 L562
  constraint perpendicular L567 L612
  constraint perpendicular L513 L567
  constraint perpendicular L481 L543
  constraint perpendicular L505 L543
  constraint perpendicular L286 L505
  constraint perpendicular L279 L286
  constraint perpendicular L434 L505
  constraint perpendicular L205 L434
  constraint perpendicular L60 L205
  constraint perpendicular L22 L60
  constraint perpendicular L22 L39
  constraint perpendicular L39 L41
  constraint perpendicular L41 L74
  constraint perpendicular L62 L74
  constraint perpendicular L62 L76
  constraint perpendicular L49 L76
  constraint parallel L409 L448
  constraint perpendicular L311 L612
  constraint perpendicular L311 L577
  constraint perpendicular L350 L577
  constraint perpendicular L350 L617
  constraint perpendicular L575 L617
  constraint perpendicular L251 L575
  constraint perpendicular L251 L322
  constraint perpendicular L274 L322
  constraint perpendicular L274 L594
  constraint perpendicular L94 L594
  constraint perpendicular L274 L465
  constraint perpendicular L138 L465
  constraint perpendicular L138 L427
  constraint perpendicular L118 L427
  constraint perpendicular L118 L552
  constraint perpendicular L472 L552
  constraint perpendicular L472 L480
  constraint perpendicular L315 L480
  constraint perpendicular L414 L505
  constraint perpendicular L300 L414
  constraint perpendicular L300 L598
  constraint perpendicular L598 L609
  constraint perpendicular L609 L623
  constraint perpendicular L566 L623
  constraint perpendicular L327 L566
  constraint perpendicular L327 L340
  constraint perpendicular L340 L362
  constraint perpendicular L309 L327
  constraint perpendicular L287 L309
  constraint perpendicular L245 L287
  constraint perpendicular L245 L402
  constraint perpendicular L218 L287
  constraint perpendicular L218 L398
  constraint perpendicular L255 L287
  constraint perpendicular L204 L255
  constraint perpendicular L204 L305
  constraint perpendicular L273 L305
  constraint perpendicular L354 L505
  constraint perpendicular L354 L556
  constraint perpendicular L288 L305
  constraint perpendicular L280 L288
  constraint perpendicular L305 L604
  constraint perpendicular L604 L618
  constraint perpendicular L305 L631
  constraint perpendicular L631 L634
  constraint perpendicular L337 L347
  constraint perpendicular L209 L410
  constraint perpendicular L222 L410
  constraint perpendicular L71 L222
  constraint perpendicular L288 L495
  constraint perpendicular L281 L637
  constraint perpendicular L636 L637
  constraint perpendicular L285 L636
  constraint perpendicular L285 L564
  constraint perpendicular L564 L587
  constraint perpendicular L396 L587
  constraint perpendicular L119 L564
  constraint perpendicular L408 L587
  constraint perpendicular L200 L564
  constraint perpendicular L32 L587
  constraint perpendicular L32 L203
  constraint perpendicular L195 L203
  constraint perpendicular L32 L38
  constraint perpendicular L203 L518
  constraint perpendicular L32 L503
  constraint perpendicular L203 L549
  constraint perpendicular L32 L605
  constraint perpendicular L203 L284
  constraint perpendicular L32 L359
  constraint perpendicular L203 L489
  constraint perpendicular L32 L641
  constraint perpendicular L528 L641
  constraint perpendicular L32 L418
  constraint perpendicular L458 L641
  constraint perpendicular L561 L596
  constraint perpendicular L418 L614
  constraint perpendicular L177 L561
  constraint perpendicular L418 L425
  constraint perpendicular L561 L590
  constraint perpendicular L418 L486
  constraint perpendicular L378 L561
  constraint perpendicular L317 L418
  constraint perpendicular L317 L368
  constraint perpendicular L418 L430
  constraint perpendicular L317 L521
  constraint perpendicular L211 L521
  constraint perpendicular L211 L224
  constraint perpendicular L339 L521
  constraint perpendicular L263 L339
  constraint perpendicular L370 L521
  constraint perpendicular L323 L414
  constraint perpendicular L239 L300
  constraint perpendicular L239 L656
  constraint perpendicular L231 L656
  constraint perpendicular L239 L664
  constraint perpendicular L346 L664
  constraint perpendicular L266 L346
  constraint perpendicular L266 L401
  constraint perpendicular L365 L401
  constraint perpendicular L365 L374
  constraint perpendicular L353 L401
  constraint perpendicular L312 L495
  constraint perpendicular L381 L567
  constraint perpendicular L333 L567
  constraint perpendicular L307 L641
  constraint perpendicular L328 L489
  constraint perpendicular L344 L608
  constraint perpendicular L598 L616
  constraint perpendicular L98 L344
  constraint perpendicular L98 L165
  constraint perpendicular L165 L571
  constraint perpendicular L147 L571
  constraint perpendicular L97 L165
  constraint perpendicular L453 L531
  constraint perpendicular L147 L493
  constraint perpendicular L158 L531
  constraint perpendicular L381 L635
  constraint perpendicular L293 L381
  constraint perpendicular L293 L393
  constraint perpendicular L369 L381
  constraint perpendicular L369 L388
  constraint perpendicular L319 L393
  constraint perpendicular L254 L319
  constraint perpendicular L254 L268
  constraint perpendicular L268 L397
  constraint perpendicular L371 L397
  constraint perpendicular L325 L371
  constraint perpendicular L397 L506
  constraint perpendicular L500 L506
  constraint perpendicular L397 L450
  constraint perpendicular L141 L506
  constraint perpendicular L397 L559
  constraint perpendicular L133 L559
  constraint perpendicular L133 L509
  constraint perpendicular L516 L559
  constraint perpendicular L133 L167
  constraint perpendicular L167 L417
  constraint perpendicular L417 L595
  constraint perpendicular L302 L595
  constraint perpendicular L332 L388
  constraint perpendicular L94 L114
  constraint perpendicular L114 L290
  constraint perpendicular L290 L456
  constraint perpendicular L114 L421
  constraint perpendicular L290 L532
  constraint perpendicular L114 L172
  constraint perpendicular L290 L511
  constraint perpendicular L114 L436
  constraint perpendicular L290 L431
  constraint perpendicular L114 L166
  constraint perpendicular L290 L534
  constraint perpendicular L114 L468
  constraint perpendicular L154 L290
  constraint perpendicular L154 L259
  constraint perpendicular L290 L551
  constraint perpendicular L154 L622
  constraint perpendicular L290 L550
  constraint perpendicular L550 L615
  constraint perpendicular L290 L600
  constraint perpendicular L432 L550
  constraint perpendicular L161 L290
  constraint perpendicular L114 L630
  constraint perpendicular L290 L454
  constraint perpendicular L320 L454
  constraint perpendicular L613 L630
  constraint perpendicular L454 L510
  constraint perpendicular L535 L630
  constraint perpendicular L253 L454
  constraint perpendicular L620 L630
  constraint perpendicular L299 L620
  constraint perpendicular L299 L508
  constraint perpendicular L526 L620
  constraint perpendicular L526 L651
  constraint perpendicular L492 L651
  constraint perpendicular L416 L526
  constraint perpendicular L174 L651
  constraint perpendicular L441 L526
  constraint perpendicular L173 L441
  constraint perpendicular L127 L173
  constraint perpendicular L127 L419
  constraint perpendicular L173 L512
  constraint perpendicular L127 L142
  constraint perpendicular L110 L173
  constraint perpendicular L127 L415
  constraint perpendicular L173 L517
  constraint perpendicular L161 L522
  constraint perpendicular L269 L419
  constraint perpendicular L431 L469
  constraint perpendicular L95 L469
  constraint perpendicular L269 L533
  constraint perpendicular L469 L547
  constraint perpendicular L114 L639
  constraint perpendicular L267 L469
  constraint perpendicular L269 L560
  constraint parallel L95 L632
  constraint perpendicular L565 L632
  constraint perpendicular L565 L602
  constraint perpendicular L602 L628
  constraint perpendicular L565 L601
  constraint perpendicular L548 L602
  constraint perpendicular L548 L597
  constraint perpendicular L597 L610
  constraint perpendicular L580 L639
  constraint perpendicular L294 L526
  constraint perpendicular L524 L547
  constraint perpendicular L568 L590
  constraint perpendicular L515 L535
  constraint perpendicular L261 L590
  constraint perpendicular L334 L627
  constraint vertical L501
  constraint coincident L546.end L501
  constraint perpendicular L501 L546
  constraint perpendicular L519 L546
  constraint perpendicular L519 L545
  constraint perpendicular L545 L582
  constraint perpendicular L476 L582
  constraint perpendicular L272 L476
  constraint perpendicular L272 L483
  constraint perpendicular L296 L665
  constraint perpendicular L91 L665
  constraint perpendicular L131 L290
  constraint perpendicular L150 L456
  constraint perpendicular L115 L290
  constraint perpendicular L91 L463
  constraint perpendicular L131 L429
  constraint perpendicular L423 L429
  constraint perpendicular L131 L163
  constraint perpendicular L163 L471
  constraint perpendicular L170 L471
  constraint perpendicular L91 L125
  constraint perpendicular L96 L125
  constraint perpendicular L91 L464
  constraint perpendicular L99 L125
  constraint perpendicular L91 L447
  constraint perpendicular L125 L168
  constraint perpendicular L91 L155
  constraint perpendicular L125 L435
  constraint perpendicular L91 L105
  constraint perpendicular L125 L466
  constraint perpendicular L113 L455
  constraint perpendicular L93 L178
  constraint perpendicular L178 L445
  constraint perpendicular L108 L171
  constraint perpendicular L108 L164
  constraint perpendicular L111 L164
  constraint perpendicular L111 L428
  constraint perpendicular L164 L459
  constraint perpendicular L438 L459
  constraint perpendicular L112 L139
  constraint perpendicular L459 L461
  constraint perpendicular L160 L164
  constraint horizontal L185
  constraint vertical L644
  constraint horizontal L696
  constraint vertical L646
  constraint coincident P0 L23.start
  constraint coincident L206.end L646
  constraint coincident L23.end L646
  constraint perpendicular L34 L646
  constraint perpendicular L34 L48
  constraint perpendicular L390 L646
  constraint perpendicular L31 L390
  constraint perpendicular L31 L201
  constraint perpendicular L201 L220
  constraint perpendicular L64 L220
  constraint perpendicular L201 L246
  constraint coincident L192.start L185
  constraint perpendicular L246 L356
  constraint perpendicular L192 L283
  constraint perpendicular L192 L210
  constraint perpendicular L210 L264
  constraint perpendicular L192 L389
  constraint perpendicular L372 L389
  constraint perpendicular L355 L372
  constraint perpendicular L185 L467
  constraint perpendicular L574 L646
  constraint perpendicular L574 L654
  constraint perpendicular L308 L654
  constraint perpendicular L308 L387
  constraint perpendicular L375 L654
  constraint perpendicular L375 L403
  constraint perpendicular L336 L403
  constraint perpendicular L208 L336
  constraint perpendicular L341 L403
  constraint perpendicular L34 L65
  constraint perpendicular L42 L65
  constraint perpendicular L34 L44
  constraint perpendicular L44 L244
  constraint perpendicular L244 L599
  constraint perpendicular L599 L629
  constraint perpendicular L592 L629
  constraint perpendicular L542 L599
  constraint perpendicular L457 L542
  constraint perpendicular L589 L599
  constraint perpendicular L34 L502
  constraint perpendicular L584 L646
  constraint perpendicular L34 L440
  constraint perpendicular L462 L646
  constraint perpendicular L34 L491
  constraint perpendicular L424 L646
  constraint perpendicular L34 L426
  constraint perpendicular L107 L646
  constraint perpendicular L34 L145
  constraint coincident L507.end L646
  constraint perpendicular L507 L646
  constraint perpendicular L34 L420
  constraint perpendicular L61 L646
  constraint perpendicular L34 L214
  constraint perpendicular L249 L646
  constraint perpendicular L34 L53
  constraint perpendicular L240 L646
  constraint perpendicular L34 L215
  constraint perpendicular L26 L646
  constraint perpendicular L26 L69
  constraint perpendicular L250 L646
  constraint perpendicular L26 L243
  constraint perpendicular L342 L646
  constraint perpendicular L26 L233
  constraint perpendicular L199 L646
  constraint perpendicular L26 L193
  constraint perpendicular L316 L646
  constraint perpendicular L26 L120
  constraint perpendicular L529 L646
  constraint perpendicular L26 L135
  constraint perpendicular L449 L646
  constraint perpendicular L26 L663
  constraint perpendicular L258 L646
  constraint perpendicular L26 L360
  constraint perpendicular L295 L646
  constraint perpendicular L26 L343
  constraint perpendicular L352 L646
  constraint perpendicular L26 L236
  constraint perpendicular L395 L646
  constraint perpendicular L26 L202
  constraint perpendicular L51 L646
  constraint perpendicular L26 L494
  constraint perpendicular L555 L646
  constraint perpendicular L26 L159
  constraint perpendicular L169 L646
  constraint perpendicular L26 L557
  constraint perpendicular L130 L646
  constraint perpendicular L26 L477
  constraint perpendicular L137 L646
  constraint perpendicular L26 L578
  constraint perpendicular L162 L646
  constraint perpendicular L26 L443
  constraint perpendicular L176 L646
  constraint perpendicular L26 L473
  constraint perpendicular L444 L646
  constraint perpendicular L26 L514
  constraint perpendicular L420 L437
  constraint coincident L217.end L185
  constraint coincident L57.start L185
  constraint perpendicular L57 L589
  constraint perpendicular L57 L358
  constraint perpendicular L358 L367
  constraint perpendicular L57 L324
  constraint perpendicular L358 L638
  constraint perpendicular L57 L257
  constraint perpendicular L357 L358
  constraint perpendicular L57 L252
  constraint perpendicular L331 L358
  constraint perpendicular L57 L380
  constraint perpendicular L449 L544
  constraint perpendicular L57 L569
  constraint perpendicular L433 L449
  constraint perpendicular L57 L537
  constraint perpendicular L449 L474
  constraint perpendicular L57 L570
  constraint perpendicular L449 L485
  constraint perpendicular L57 L523
  constraint coincident L50.start L185
  constraint perpendicular L185 L504
  constraint vertical L36
  constraint perpendicular L30 L36
  constraint perpendicular L30 L640
  constraint perpendicular L446 L640
  constraint perpendicular L446 L478
  constraint perpendicular L478 L520
  constraint perpendicular L488 L520
  constraint perpendicular L488 L525
  constraint perpendicular L525 L588
  constraint perpendicular L411 L488
  constraint perpendicular L391 L411
  constraint perpendicular L277 L391
  constraint perpendicular L260 L277
  constraint perpendicular L260 L270
  constraint perpendicular L270 L314
  constraint perpendicular L260 L606
  constraint perpendicular L194 L270
  constraint perpendicular L194 L585
  constraint perpendicular L36 L88
  constraint horizontal L81
  constraint perpendicular L56 L81
  constraint coincident L80.start L185
  constraint perpendicular L80 L185
  constraint coincident L86.end L185
  constraint perpendicular L86 L185
  constraint horizontal L37
  constraint parallel L37 L78
  constraint perpendicular L84 L87
  constraint perpendicular L77 L81
  constraint perpendicular L77 L79
  constraint perpendicular L79 L298
  constraint perpendicular L235 L298
  constraint perpendicular L66 L235
  constraint perpendicular L298 L497
  constraint perpendicular L497 L554
  constraint perpendicular L298 L385
  constraint perpendicular L297 L497
  constraint perpendicular L298 L304
  constraint perpendicular L151 L304
  constraint perpendicular L151 L382
  constraint perpendicular L228 L382
  constraint coincident L50.end L185
  constraint perpendicular L88 L132
  constraint perpendicular L103 L132
  constraint perpendicular L103 L128
  constraint perpendicular L132 L148
  constraint perpendicular L148 L157
  constraint perpendicular L132 L140
  constraint perpendicular L140 L152
  constraint perpendicular L129 L132
  constraint perpendicular L140 L442
  constraint perpendicular L15 L56
  constraint perpendicular L19 L81
  constraint perpendicular L56 L702
  constraint perpendicular L20 L81
  constraint perpendicular L56 L182
  constraint perpendicular L17 L81
  constraint perpendicular L21 L56
  constraint perpendicular L11 L81
  constraint perpendicular L6 L56
  constraint perpendicular L81 L189
  constraint perpendicular L9 L56
  constraint perpendicular L81 L180
  constraint perpendicular L56 L149
  constraint perpendicular L149 L661
  constraint perpendicular L661 L668
  constraint perpendicular L92 L149
  constraint perpendicular L128 L643
  constraint coincident L134.start L185
  constraint perpendicular L185 L650
  constraint perpendicular L185 L655
  constraint perpendicular L90 L650
  constraint perpendicular L185 L648
  constraint perpendicular L143 L650
  constraint perpendicular L8 L185
  constraint perpendicular L7 L650
  constraint perpendicular L185 L692
  constraint perpendicular L650 L672
  constraint perpendicular L5 L185
  constraint perpendicular L650 L697
  constraint perpendicular L10 L185
  constraint perpendicular L181 L650
  constraint perpendicular L4 L185
  constraint perpendicular L4 L18
  constraint perpendicular L12 L18
  constraint perpendicular L4 L184
  constraint perpendicular L13 L184
  constraint perpendicular L4 L698
  constraint perpendicular L14 L698
  constraint perpendicular L4 L186
  constraint perpendicular L186 L187
  constraint perpendicular L4 L699
  constraint perpendicular L652 L699
  constraint perpendicular L439 L652
  constraint perpendicular L175 L439